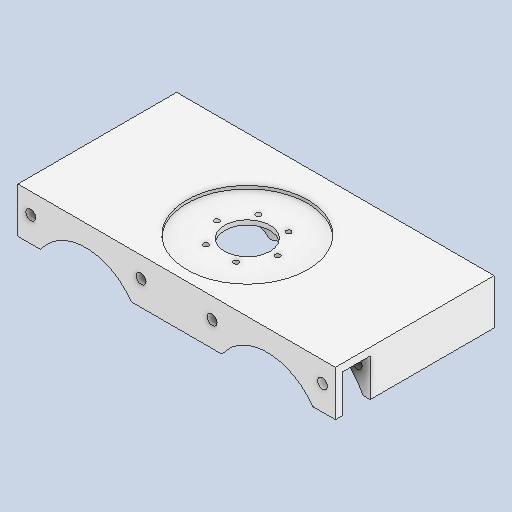
# Autodesk Inventor part: motor_holder
Saved by Autodesk Inventor 2025.3 (Build 293356030, 356C)
## iProperties
Created: 2025-09-14
Part Number: motor_holder
Material: PLA+ filament
Document SubType Name: Modeling
Designer: MSI
Mass: 263.891 g
Surface Area: 706.305 cm^2
Volume: 214.545 cm^3
Density: 1.23 g/cm^3
Appearance: 일반
Author: MSI
Autodesk Inventor part; units mm, degrees
ref_plane "YZ Plane" through (0, 0, 0) normal (1, 0, 0) x (0, 1, 0)
ref_plane "XZ Plane" through (0, 0, 0) normal (0, 1, 0) x (-1, 0, 0)
ref_plane "XY Plane" through (0, 0, 0) normal (0, 0, 1) x (1, 0, 0)
sketch "스케치1" plane through (0, 0, 0) normal (0, 0, 1) x (1, 0, 0)
  line L0 (105, 15) -> (-105, 15)
  line L1 (-105, 15) -> (-105, -15)
  line L2 (-105, -15) -> (105, -15)
  line L3 (105, -15) -> (105, 15)
  line L4 (105, 15) -> (-105, -15) construction
  line L5 (-105, 15) -> (105, -15) construction
  point P0 (0, 0)
  dimension "d0" = 210
  dimension "d1" = 30
  constraints: 12 end point, 2 midpoint, 2 parallel, 1 horizontal, 1 perpendicular
  measures "d0" distance of L2.end L1.end
  measures "d1" distance of L1.end L0.end
extrude "돌출1" add sketch "스케치1" along normal mid plane 100
sketch "스케치2" plane through (0, 0, 50) normal (0, 0, 1) x (1, 0, 0)
  line L0 (105, 15) -> (-105, 15) projected
  circle A0 centre (-60, -35) radius 45
  circle A1 centre (60, -35) radius 45
  point P0 (0, 0)
  point P1 (0, -35)
  dimension "d35" = 90
  dimension "d36" = 90
  dimension "d37" = 50
  dimension "d38" = 120
  dimension "d39" = 60
  constraints: 2 centre point, 1 horizontal alignment, 1 vertical alignment
  measures "d35" diameter of A0
  measures "d36" diameter of A1
  measures "d37" distance from line of L0 A0.centre
  measures "d38" distance of A1.centre A0.centre
  measures "d39" horizontal distance of point (0, 0) A0.centre
extrude "돌출2" cut sketch "스케치2" against normal blind 100
sketch "스케치3" plane through (0, 0, 50) normal (0, 0, 1) x (1, 0, 0)
  line L0 (-105, -15) -> (105, -15)
  line L1 (105, -15) -> (105, 10)
  line L2 (105, 10) -> (-105, 10)
  line L3 (-105, 10) -> (-105, -15)
  line L4 (105, 15) -> (-105, 15) projected
  line L5 (-105, 15) -> (-105, -15) projected
  line L6 (-105, -15) -> (105, -15) projected
  point P0 (0, 0)
  point P1 (0, 10)
  point P2 (100.3113, -15)
  dimension "d9" = 5
  constraints: 8 end point, 2 collinear, 2 parallel, 1 horizontal, 1 midpoint, 1 perpendicular, 1 vertical alignment
  measures "d9" distance between parallel lines of L2 L4
extrude "돌출3" cut sketch "스케치3" against normal blind 18
sketch "스케치4" plane through (-105, 15, 50) normal (0, 1, 0) x (1, 0, 0)
  circle A0 centre (105, 41.75) radius 40
  line L0 (210, 0) -> (0, 0) projected
  point P0 (105, 50)
  dimension "d13" = 80
  dimension "d14" = 41.75
  constraints: 1 centre point, 1 vertical alignment
  measures "d13" diameter of A0
  measures "d14" distance from line of L0 A0.centre
extrude "돌출4" cut sketch "스케치4" against normal blind 2
sketch "스케치8" plane through (-19.6887, -15, -50) normal (0, -1, 0) x (1, 0, 0)
  circle A0 centre (19.6887, 58.25) radius 40 projected
  point P0 (19.6887, 50)
  constraints: 1 coincident
hole "구멍4" at (0, -15, 8.25) direction (0, 1, 0) diameter 30 end through all counterbore diameter 80 counterbore depth 25
sketch "스케치14" plane through (0, 0, 50) normal (0, 0, 1) x (1, 0, 0)
  line L0 (105, 15) -> (105, -15) projected
  line L1 (-105, 15) -> (105, 15)
  line L2 (105, 15) -> (105, -15)
  line L3 (105, -15) -> (-105, -15)
  line L4 (-105, -15) -> (-105, 15)
  point P0 (0, 0)
  constraints: 8 end point, 2 parallel, 1 horizontal, 1 perpendicular
extrude "돌출6" add sketch "스케치14" along normal blind 5
sketch "스케치15" plane through (0, 0, 50) normal (0, 0, -1) x (-1, 0, 0)
  circle A0 centre (-60, -35) radius 41
  line L0 (-105, 15) -> (105, 15) projected
  line L1 (-105, -15) -> (-105, 15) projected
  line L2 (0, 15) -> (0, -71.231)
  circle A1 centre (60, -35) radius 41
  point P0 (0, 0)
  dimension "d99" = 82
  dimension "d100" = 50
  dimension "d101" = 45
  constraints: 2 centre point, 2 end point, 1 midpoint, 1 symmetric about line, 1 vertical, 1 other
  measures "d99" diameter of A0
  measures "d100" distance from line of L0 A0.centre
  measures "d101" distance from line of L1 A0.centre
extrude "돌출7" cut sketch "스케치15" against normal through all draft -45
sketch "스케치16" plane through (0, 0, 55) normal (0, 0, 1) x (1, 0, 0)
  line L0 (-96.5, 1.5) -> (-23.5, 1.5) construction
  line L1 (105, 15) -> (-105, 15) projected
  line L2 (-24.2089, -15) -> (24.2089, -15) construction
  line L3 (0, -15) -> (0, 15) construction
  line L4 (96.5, 1.5) -> (23.5, 1.5) construction
  point P0 (0, 0)
  point P1 (-60, 1.5)
  dimension "d104" = 73
  dimension "d105" = 13.5
  dimension "d113" = 120
  constraints: 6 end point, 3 midpoint, 2 symmetric about line, 1 horizontal
  measures "d104" distance of L0.start L0.end
  measures "d105" distance between parallel lines of L0 L1
  measures "d113" diameter of point (-60, 1.5) L3
hole "구멍9" at (-96.5, 1.5, 55) at (-23.5, 1.5, 55) at (23.5, 1.5, 55) at (96.5, 1.5, 55) direction (0, 0, -1) diameter 6.6 end through all clearance for "Flat Head Machine Screw" size "M6" standard "Ansi Metric M Profile"
sketch "스케치11" plane through (-105, 10, 50) normal (0, -1, 0) x (1, 0, 0)
  circle A0 centre (105, -41.75) radius 15 projected
  line L0 (105, -41.75) -> (125, -41.75) construction
  point P0 (105, -50)
  dimension "d74" = 20
  constraints: 2 end point, 1 horizontal
  measures "d74" distance of L0.start L0.end
hole "구멍7" at (20, 10, 8.25) direction (0, 1, 0) diameter 3.4 end through all clearance for "Flat Head Machine Screw" size "M3" standard "Ansi Metric M Profile"
sketch "스케치12" plane through (0, 0, -50) normal (0, 0, -1) x (-1, 0, 0)
  line L0 (-12.5, -10) -> (12.5, -10) construction
  line L1 (-19.6887, -15) -> (19.6887, -15) projected
  point P0 (0, 0)
  point P1 (0, -10)
  dimension "d83" = 5
  dimension "d84" = 25
  constraints: 2 end point, 1 horizontal, 1 midpoint, 1 vertical alignment
  measures "d83" distance between parallel lines of L1 L0
  measures "d84" distance of L0.start L0.end
sketch "스케치13" plane through (0, 0, -40) normal (0, 0, -1) x (-1, 0, 0)
  circle A0 centre (-12.5, -10) radius 1.7 projected
  circle A1 centre (-12.5, -10) radius 4.2
  circle A2 centre (12.5, -10) radius 1.7 projected
  circle A3 centre (12.5, -10) radius 4.2
  point P0 (0, 0)
  dimension "d93" = 8.4
  dimension "d94" = 8.4
  constraints: 2 centre point, 2 coincident
  measures "d93" diameter of A1
  measures "d94" diameter of A3
pattern_circular "원형 패턴1" count 6 over 360 about axis through (0, 219.5208, 8.25) along (0, -1, 0) of "구멍7"
equation "\"d94\" = d93"
